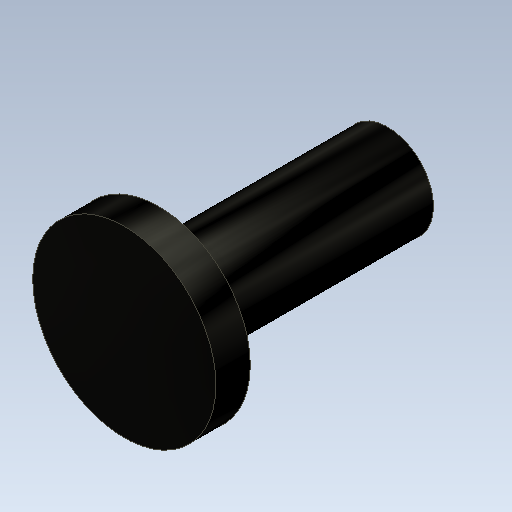
# Autodesk Inventor part: M4 六角穴付き ローヘッドキャップ (極低頭タイプ) L10
Saved by Autodesk Inventor 2020.2 (Build 242310000, 310)
## iProperties
Created: 2018-03-18
Part Number: M4 六角穴付き ローヘッドキャップ (極低頭タイプ) L10
Material: 鋼、炭素鋼
Document SubType Name: Modeling
Designer: Takumi
Density: 7.85 g/cm^3
Appearance: ガンメタル
Mass: 1.57834 g
Surface Area: 2.63894 cm^2
Volume: 0.201062 cm^3
Author: Takumi
Autodesk Inventor part; units mm, degrees
ref_plane "YZ Plane" through (0, 0, 0) normal (1, 0, 0) x (0, 1, 0)
ref_plane "XZ Plane" through (0, 0, 0) normal (0, 1, 0) x (-1, 0, 0)
ref_plane "XY Plane" through (0, 0, 0) normal (0, 0, 1) x (1, 0, 0)
sketch "スケッチ1" plane through (0, 0, 0) normal (0, 0, 1) x (1, 0, 0)
  circle A0 centre (0, 0) radius 4
  circle A1 centre (0, 0) radius 2
  dimension "d0" = 8
  dimension "d1" = 4
  constraints: 2 centre point, 2 coincident
  measures "d0" diameter of A0
  measures "d1" diameter of A1
extrude "押し出し1" add sketch "スケッチ1" along normal blind 1.5 contours A0 | A1
extrude "押し出し2" add sketch "スケッチ1" against normal blind 10 contours A1
